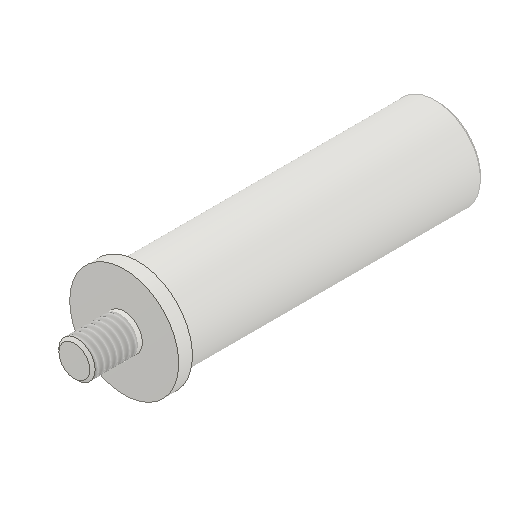
# Autodesk Inventor part: Compensador Haste
Saved by Autodesk Inventor 2026.1 (Build 301233020, 233B)
## iProperties
Company: Elgin
Created: 2025-10-02
Part Number: Compensador Haste
Material: Aço SAE 1045
Document SubType Name: Modeling
Designer: Willian Pinheiro
Mass: 19.89 g
Surface Area: 16.129 cm^2
Volume: 2.53375 cm^3
Density: 7.85 g/cm^3
Appearance: Aço
Description: Compensador Haste
Dimensões: Ø12 x 40 mm
Total: 4
Author: Willian Pinheiro
Title: Testador Controle
Revision Number: 00
Autodesk Inventor part; units mm, degrees
ref_plane "YZ Plane" through (0, 0, 0) normal (1, 0, 0) x (0, 1, 0)
ref_plane "XZ Plane" through (0, 0, 0) normal (0, 1, 0) x (-1, 0, 0)
ref_plane "XY Plane" through (0, 0, 0) normal (0, 0, 1) x (1, 0, 0)
sketch "Esboço1" plane through (0, 0, 0) normal (0, 0, 1) x (1, 0, 0)
  line L0 (-7.2, 0) -> (1.2, 0) construction
  line L1 (0, -13.5) -> (0, 42.5) construction
  line L2 (0, 34.5) -> (0, -5.5)
  line L3 (0, -5.5) -> (-2, -5.5)
  line L4 (-2, -5.5) -> (-2, 0)
  line L5 (-2, 0) -> (-6, 0)
  line L6 (-6, 0) -> (-6, 1.5)
  line L7 (-6, 1.5) -> (-5, 1.5)
  line L8 (-5, 1.5) -> (-5, 34.5)
  line L9 (-5, 34.5) -> (0, 34.5)
  point P0 (0, 0)
  dimension "d0" = 10
  dimension "d1" = 12
  dimension "d2" = 1.5
  dimension "d3" = 5.5
  dimension "d4" = 33
  dimension "d7" = 4
  dimension "d21" = 40
  constraints: 16 end point, 6 perpendicular, 2 collinear, 1 horizontal, 1 vertical
  measures "d0" diameter of L8 L1
  measures "d1" diameter of L6 L1
  measures "d2" distance of L5.end L6.end
  measures "d3" distance of L3.end L4.end
  measures "d4" distance of L7.end L8.end
  measures "d7" diameter of L4 L1
  measures "d21" distance between parallel lines of L9 L3
revolve "Revolução1" add sketch "Esboço1" angle 360 about axis through (0, -10, 0) along (0, 1, 0)
sketch "Esboço2" plane through (0, 34.5, 0) normal (0, 1, 0) x (1, 0, 0)
  circle A0 centre (0, 0) radius 5 projected
  constraints: 1 coincident
hole "Furo1" at (0, 34.5, 0) direction (0, -1, 0) diameter 4.917 depth 15 tip angle 118 thread size "M6x1" class "6H" standard "ISO Metric profile"
thread "Rosca1" size "M4x0.7" class "6g" standard "ANSI Metric M Profile" length 5
chamfer "Chanfro1" distance 0.3 angle 45 3 edges at (2, -5.5, 0) (5, 34.5, 0) (0, 34.5, -2.4585)
